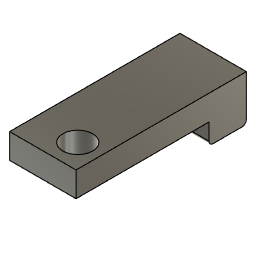
limitSW_guide v1 (Autodesk Fusion 360 design; units mm, degrees)
Autodesk Fusion 360 part; units mm, degrees
sketch "Sketch1" plane through (0, 0, 0) normal (0, 0, 1) x (1, 0, 0)
  line L0 (0, 0) -> (8, 0)
  line L1 (8, 0) -> (8, 16)
  line L2 (8, 16) -> (0, 16)
  line L3 (0, 16) -> (0, 0)
  circle A0 centre (5.2273, 2.9759) radius 1.8
  dimension "d1" = 8
  dimension "d2" = 16
  dimension "d3" = 3.6
  constraint horizontal L0
  constraint vertical L1
  constraint horizontal L2
  constraint vertical L3
  constraint coincident L0.start L3.end
  measures "d1" distance of L0.start L0.end
  measures "d2" distance of L0.start L2.end
  measures "d3" diameter of A0
extrude "Extrude1" add sketch "Sketch1" along normal blind 3
sketch "Sketch2" plane through (0, 16, 0) normal (0, 1, 0) x (-1, 0, 0)
  line L0 (-8, 0) -> (0, 0)
  line L1 (0, 0) -> (0, 3)
  line L2 (0, 3) -> (-8, 3)
  line L3 (-8, 3) -> (-8, 0)
  line L4 (-8, 3) -> (-1, 3)
  line L5 (-1, 3) -> (-1, -2.5)
  line L6 (-1, -2.5) -> (-8, -2.5)
  line L7 (-8, -2.5) -> (-8, 3)
  dimension "d7" = 7
  dimension "d8" = 5.5
  constraint horizontal L4
  constraint vertical L5
  constraint horizontal L6
  constraint vertical L7
  constraint coincident L2.end L3.start
  measures "d7" distance of L2.end L4.end
  measures "d8" distance of L2.end L6.end
extrude "Extrude2" add sketch "Sketch2" along normal blind 4.5 contours L0 L2 L3 L4 L5 L7 | L0 L5 L6 L7
move_face "OffsetFaces1" offset 1 1 faces at (1, 19, 0.1667)
fillet "Fillet1" radius 0.5 2 edges at (4, 20.5, -2.5) (4, 16, -2.5)
